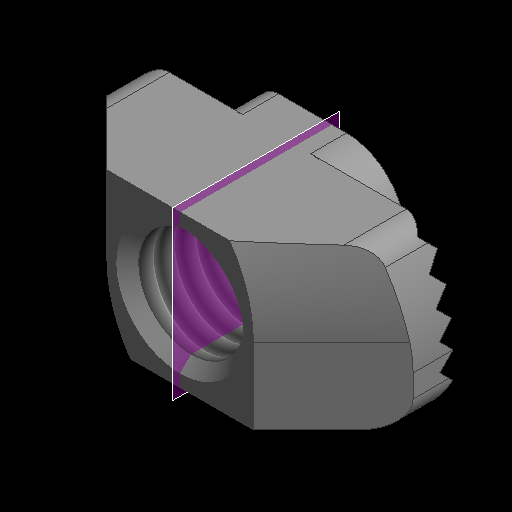
# Autodesk Inventor part: 14162_m
Saved by Autodesk Inventor 2022 (Build 260153000, 153)
## iProperties
Category: PARTsolutions
Company: 8020
Part Number: 14162_m
Material: Generic
Catalog Web Link: www.cadenas.de
Description: 14162, 14164, 14166, 13118, 13111, 13113, 13115, 13117, 13112, 13110, 13114, 13116, 13119, 14165, 13123, 13127, 13129, 13132, 13122, 13120, 13124, 13130, 13133, 13121, 13125_m-Drop-In T-Nuts
Vendor: 8020
Document SubType Name: Modeling
Designer: partserver
Manufacturer: 8020
Mass: 0.188208 g
Surface Area: 3.11076 cm^2
Volume: 0.188208 cm^3
Density: 1 g/cm^3
Appearance: PSOLRGB-175-175-175
PSOL_IDENT_0: {$CADENAS_DATA\23d-libs\8020\metric\fastening_options\14162_m.prj},326 {VTYP=3D},{NB=14162_m},{LINA=
PSOL_IDENT_1: 14162},{NN=14162, 14164, 14166, 13118, 13111, 13113, 13115, 13117, 13112, 13110, 13114, 13116, 13119
PSOL_IDENT_2: , 14165, 13123, 13127, 13129, 13132, 13122, 13120, 13124, 13130, 13133, 13121, 13125_m},{DATE=31.07.
PSOL_IDENT_3: 2020 09:21:26},{GEOMDATE=09.09.2015 07:46:58},{VERSION=},{LINEID=10},{WBVAR=MAT,A},{WBNUMERIC=}  {NB=
PSOL_IDENT_4: 14162_m},{LINA=14162},{KT=DUMMY},{PN=14162},{MAT=1},{MAT1= '1','Steel','2','Stainless Steel' },{A=10
PSOL_IDENT_5: -32},{AALG= '10-32','10-32','M4','M4' },{A1=0.1900},{B=11.50},{C=5.70},{D=4.50},{E=1.20},{F=5.50},{W=
PSOL_IDENT_6: .0012},{CC=6-10, 6-25},{NO=1},{TT=UNF}
NB: 14162_m
NN: 14162, 14164, 14166, 13118, 13111, 13113, 13115, 13117, 13112, 13110, 13114, 13116, 13119, 14165, 13123, 13127, 13129, 13132, 13122, 13120, 13124, 13130, 13133, 13121, 13125_m
NT: Drop-In T-Nuts
NBSYN: $PN._m
LINA: 14162
CATALOG: 80/20
PN: 14162
MAT: Steel
A: 10-32
B: 11.5
C: 5.7
D: 4.5
E: 1.2
F: 5.5
W: .0012
CC: 6-10, 6-25
SUPPLIER: 8020
ARTICLENO: 14162_m
BOMINFO: 14162
CREATOR: CADENAS GmbH
Title: 14162
Author: Cadenas PARTsolutions
Comments: Drop-In T-Nuts
Autodesk Inventor part; units mm, degrees
sketch "Sketch_1" plane through (0, 0, 0) normal (0, 1, 0) x (-1, 0, 0)
  arc A0 (5.75, 1.85) -> (4.75, 2.85) centre (4.75, 1.85) ccw
  line L0 (4.75, 2.85) -> (-4.1436, 2.85)
  arc A1 (-4.1436, 2.85) -> (-5.0569, 2.2571) centre (-4.1436, 1.85) ccw
  arc A2 (-5.0569, 2.2571) -> (-5.75, -1) centre (2.25, -1) ccw
  line L1 (-5.75, -1) -> (-5.75, -1.85)
  arc A3 (-5.75, -1.85) -> (-4.75, -2.85) centre (-4.75, -1.85) ccw
  line L2 (-4.75, -2.85) -> (4.1436, -2.85)
  arc A4 (4.1436, -2.85) -> (5.0569, -2.2571) centre (4.1436, -1.85) ccw
  arc A5 (5.0569, -2.2571) -> (5.75, 1) centre (-2.25, 1) ccw
  line L3 (5.75, 1) -> (5.75, 1.85)
  constraints: 12 point on circle, 8 end point, 6 centre point
extrude "Extrusion1" add sketch "Sketch_1" along normal blind 5.7
sketch "Sketch_2" plane through (0, 0, 0) normal (1, 0, 0) x (0, 1, 0)
  line L0 (6, 4) -> (4.5, 4)
  line L1 (4.5, 4) -> (4, 3.5)
  line L2 (4, 3.5) -> (4.5, 3)
  line L3 (4.5, 3) -> (4, 2.5)
  line L4 (4, 2.5) -> (4.5, 2)
  line L5 (4.5, 2) -> (4, 1.5)
  line L6 (4, 1.5) -> (4.5, 1)
  line L7 (4.5, 1) -> (4, 0.5)
  line L8 (4, 0.5) -> (4.5, 0)
  line L9 (4.5, 0) -> (4, -0.5)
  line L10 (4, -0.5) -> (4.5, -1)
  line L11 (4.5, -1) -> (4, -1.5)
  line L12 (4, -1.5) -> (4.5, -2)
  line L13 (4.5, -2) -> (4, -2.5)
  line L14 (4, -2.5) -> (4.5, -3)
  line L15 (4.5, -3) -> (4, -3.5)
  line L16 (4, -3.5) -> (4.5, -4)
  line L17 (4.5, -4) -> (6, -4)
  line L18 (6, -4) -> (6, 4)
  constraints: 38 end point
extrude "Extrusion2" cut sketch "Sketch_2" along normal mid plane 11.5
sketch "Sketch_3" plane through (0, 0, 0) normal (0, 0, 1) x (1, 0, 0)
  line L0 (-6.75, 4) -> (-6.75, -1)
  line L1 (-6.75, -1) -> (6.75, -1)
  line L2 (6.75, -1) -> (6.75, 4)
  line L3 (6.75, 4) -> (2.75, 0)
  line L4 (2.75, 0) -> (-2.75, 0)
  line L5 (-2.75, 0) -> (-6.75, 4)
  constraints: 12 end point
extrude "Extrusion3" cut sketch "Sketch_3" along normal mid plane 5.7
sketch "Sketch_4" plane through (0, 0, 0) normal (0, 0, 1) x (1, 0, 0)
  line L0 (-2.25, -1) -> (-2.25, 3)
  line L1 (-2.25, 0) -> (2.75, 0)
  line L2 (2.75, 0) -> (5.75, 3)
  line L3 (5.75, 3) -> (6.75, 3)
  line L4 (6.75, 3) -> (6.75, -1)
  line L5 (6.75, -1) -> (-2.25, -1)
  line L6 (-2.25, -1) -> (-2.25, 0)
  constraints: 14 end point
revolve "Revolution1" cut sketch "Sketch_4" angle 60 about axis through (-2.25, -1, 0) along (0, -1, 0)
sketch "Sketch_5" plane through (0, 0, 0) normal (0, 0, 1) x (1, 0, 0)
  line L0 (2.25, 3) -> (2.25, -1)
  line L1 (2.25, -1) -> (-6.75, -1)
  line L2 (-6.75, -1) -> (-6.75, 3)
  line L3 (-6.75, 3) -> (-5.75, 3)
  line L4 (-5.75, 3) -> (-2.75, 0)
  line L5 (-2.75, 0) -> (2.25, 0)
  line L6 (2.25, 0) -> (2.25, -1)
  constraints: 14 end point
revolve "Revolution2" cut sketch "Sketch_5" angle 60 about axis through (2.25, 3, 0) along (0, -1, 0)
sketch "Sketch_6" plane through (0, 3.6, 0) normal (0, 1, 0) x (1, 0, 0)
  arc A0 (-2.75, -2.1) -> (-2, -2.85) centre (-2, -2.1) ccw
  line L0 (-2, -2.85) -> (0.55, -2.85)
  arc A1 (0.55, -2.85) -> (2.75, -0.65) centre (0.55, -0.65) ccw
  line L1 (2.75, -0.65) -> (2.75, 2.1)
  arc A2 (2.75, 2.1) -> (2, 2.85) centre (2, 2.1) ccw
  line L2 (2, 2.85) -> (-0.55, 2.85)
  arc A3 (-0.55, 2.85) -> (-2.75, 0.65) centre (-0.55, 0.65) ccw
  line L3 (-2.75, 0.65) -> (-2.75, -2.1)
  constraints: 8 end point, 8 point on circle, 4 centre point
extrude "Extrusion4" add sketch "Sketch_6" along normal blind 2.1
sketch "Sketch_8" plane through (0, 0, 0) normal (0, 0, 1) x (1, 0, 0)
  line L0 (0, 0) -> (0, 5.7)
  line L1 (0, 5.7) -> (2.413, 5.7)
  line L2 (2.413, 5.7) -> (1.9837, 5.2707)
  line L3 (1.9837, 5.2707) -> (1.9837, 0.4293)
  line L4 (1.9837, 0.4293) -> (2.413, 0)
  line L5 (2.413, 0) -> (0, 0)
  line L6 (0, 0) -> (0, 5.7)
  constraints: 14 end point
revolve "Revolution3" cut sketch "Sketch_8" angle 360 about axis through (0, 0, 0) along (0, -1, 0)
thread "Thread1" size "10-32 UNF" class "2B" standard "ANSI Unified Screw Threads" full length
ref_plane "1_XY" through (0, 5.7, 0) normal (0, 1, 0) x (1, 0, 0)
ref_plane "1_YZ" through (0, 5.7, 0) normal (1, 0, 0) x (0, 0, -1)
ref_plane "1_ZX" through (0, 5.7, 0) normal (0, 0, -1) x (0, 1, 0)
ref_plane "2_XY" through (0, 0, 0) normal (0, 1, 0) x (1, 0, 0)
ref_plane "2_YZ" through (0, 0, 0) normal (1, 0, 0) x (0, 0, -1)
ref_plane "2_ZX" through (0, 0, 0) normal (0, 0, -1) x (0, 1, 0)
body "Solid1"
